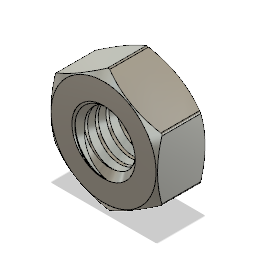
Knee Lower Pulley (Autodesk Fusion 360 archive; units mm, degrees)
design "M4 Nut v3"
Autodesk Fusion 360 part; units mm, degrees
sketch "Skizze1" plane through (0, 0, 0) normal (0, 0, 1) x (1, 0, 0)
  line L0 (-3.5, -2.0207) -> (0, -4.0415)
  line L1 (0, -4.0415) -> (3.5, -2.0207)
  line L2 (3.5, -2.0207) -> (3.5, 2.0207)
  line L3 (3.5, 2.0207) -> (0, 4.0415)
  line L4 (0, 4.0415) -> (-3.5, 2.0207)
  line L5 (-3.5, 2.0207) -> (-3.5, -2.0207)
  dimension "d3" = 3.5
  constraint vertical L5
  measures "d3" distance of origin L5
extrude "Extrusion1" add sketch "Skizze1" along normal mid plane 3.2
sketch "Skizze2" plane through (0, 0, 1.6) normal (0, 0, 1) x (1, 0, 0)
  line L0 (-3.5, 2.0207) -> (-3.5, -2.0207)
  line L1 (-3.5, -2.0207) -> (0, -4.0415)
  line L2 (0, -4.0415) -> (3.5, -2.0207)
  line L3 (3.5, -2.0207) -> (3.5, 2.0207)
  line L4 (3.5, 2.0207) -> (0, 4.0415)
  line L5 (0, 4.0415) -> (-3.5, 2.0207)
hole "Bohrung1" at (0, 0, 1.6) direction (0, 0, -1) diameter 3.332 end through all
thread "Gewinde1" "ISO Metric profile 4.0 M4x0.7 6H" major diameter 4.1095 minor diameter 3.332 pitch 0.7 angle 60 modelled right hand crest width 0.193 on face at (0.083, -1.6639, 0.5333) crest through (1.666, 0, 1.425)
sketch "Skizze4" plane through (0, 0, 0) normal (1, 0, 0) x (0, 0, -1)
  line L0 (1.6, 2.0207) -> (1.6, 4.0415)
  line L1 (1.6, -4.0415) -> (1.6, -2.0207)
  line L2 (1.6, 4.0415) -> (-1.6, 4.0415)
  line L3 (1.2536, 4.0415) -> (1.6, 3.4415)
  line L4 (1.6, 4.0415) -> (1.3402, 3.8915) construction
  line L5 (1.6, 3.4415) -> (1.6, 0)
  line L6 (1.2536, 4.0415) -> (0, 4.0415)
  line L7 (0, 1.75) -> (0, 22.5) construction
  line L8 (-1.2536, 4.0415) -> (0, 4.0415)
  line L9 (-1.2536, 4.0415) -> (-1.6, 3.4415)
  line L10 (-1.6, 3.4415) -> (-1.6, 0)
  line L11 (-1.6, 0) -> (1.6, 0)
  line L12 (-1.6, 4.6415) -> (0, 4.6415)
  line L13 (1.6, 4.6415) -> (0, 4.6415)
  line L14 (1.6, 4.6415) -> (2.2, 3.6022)
  line L15 (2.2, 3.6022) -> (2.2, -0.6)
  line L16 (-2.2, -0.6) -> (2.2, -0.6)
  line L17 (-2.2, 3.6022) -> (-2.2, -0.6)
  line L18 (-1.6, 4.6415) -> (-2.2, 3.6022)
  line L19 (-1.6, 0) -> (-2.2, 0)
  line L20 (1.6, 0) -> (2.2, 0)
  line L21 (1.6, -2.0207) -> (1.6, 2.0207)
  line L22 (-1.75, 0) -> (-22.5, 0)
  dimension "d18" = 0.3
  dimension "d19" = 0.6
  dimension "d23" = 150
  constraint coincident L2 L3.start
  constraint coincident L0 L3.end
  constraint coincident L0.end L2.start
  constraint midpoint L2 L6.end
  constraint symmetric L3.start L7 L8.start
  constraint symmetric L3.end L7 L9.end
  constraint symmetric L5.end L7 L10.end
  constraint symmetric L6.end L7 L8.end
  constraint coincident L17 L19.end
  constraint perpendicular L17 L19
  constraint coincident L15 L20.end
  constraint perpendicular L15 L20
  constraint perpendicular L3 L4
  constraint coincident L3 L4.end
  constraint vertical L10
  constraint collinear L19 L22
  measures "d18" distance of L0.end L4.end
  measures "d23" angle of L3 L5
revolve "Drehen1" cut sketch "Skizze4" angle 360 about axis through (0, 0, 1.75) along (0, 0, 1) contours L0 L2 L5 L6 L8 L9 L10 L12 L13 L14 L15 L17 L18 L19 L20 L21 L22 | L0 L2 L3
fillet "Abrundung1" radius 0.15 6 edges at (3.5, 2.0207, 0) (3.5, -2.0207, 0) (0, -4.0415, 0) (-3.5, -2.0207, 0) (0, 4.0415, 0) (-3.5, 2.0207, 0)
sketch "Skizze5" plane through (0, 0, 0) normal (1, 0, 0) x (0, 0, -1)
  line L0 (-1.6, 2.0743) -> (-1.1757, 1.65)
  line L1 (-1.1757, 1.65) -> (0, 1.65)
  line L2 (0, 1.75) -> (0, 22.5)
  line L3 (0, 1.65) -> (0, 0) construction
  line L4 (-1.1757, 1.65) -> (-1.6, 1.65) construction
  line L5 (-1.6, 1.65) -> (-1.3879, 1.8621) construction
  line L6 (-1.6, 2.0743) -> (-1.6, 0)
  line L7 (-1.6, 0) -> (0, 0)
  line L8 (1.1757, 1.65) -> (0, 1.65)
  line L9 (1.6, 2.0743) -> (1.1757, 1.65)
  line L10 (1.6, 2.0743) -> (1.6, 0)
  line L11 (1.6, 0) -> (0, 0)
  line L12 (-1.6, 3.4415) -> (-1.6, -3.4415)
  dimension "d28" = 1.65
  dimension "d29" = 0.3
  dimension "d31" = 45
  constraint horizontal L1
  constraint coincident L1.end L2
  constraint coincident L3.end L7.end
  constraint coincident L0 L5.end
  constraint perpendicular L0 L5
  constraint symmetric L0.start L2 L9.start
  constraint symmetric L0.end L2 L8.start
  constraint symmetric L1.end L2 L3.start
  constraint symmetric L2 L6.end L10.end
  constraint symmetric L2 L3.end L7.end
  constraint horizontal L7
  constraint vertical L6
  constraint horizontal L4
  constraint coincident L4.end L6
  constraint collinear L6 L12
  measures "d28" distance of L1.end L3.end
  measures "d29" distance of L4.end L5.end
  measures "d31" angle of L0 L6
revolve "Drehen2" cut sketch "Skizze5" angle 360 about axis through (0, 0, 1.75) along (0, 0, 1)
equation "HexWidth = 7 mm" comment "Side-to-side width"
equation "Height = 3.2 mm"
equation "d3 = HexWidth / 2"
equation "d4 = Height"
equation "ChamferDepth = 0.3 mm" comment "Corner chamfer depth"
equation "ChamferAngle = 30 deg" comment "Corner chamfer angle"
equation "ThreadChamferDepth = 0.3 mm"
equation "d18 = ChamferDepth"
equation "d19 = 2 * ChamferDepth"
equation "SideFillet = 0.15 mm" comment "Fillet of the sides"
equation "d22 = SideFillet"
equation "d23 = 180 deg - ChamferAngle"
equation "ThreadChamferAngle = 45 deg"
equation "CoreDrill = 3.3 mm" comment "Core drill size for the given thread. Used to compute the thread chamfer."
equation "d28 = CoreDrill / 2"
equation "d29 = ThreadChamferDepth"
equation "d31 = ThreadChamferAngle"
named bodies: "Nut"
